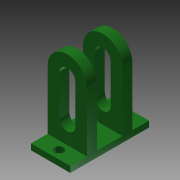
# Autodesk Inventor part: Tensioning Bracket
Saved by Autodesk Inventor 2015 SP1 (Build 190203100, 203)
## iProperties
Created: 2015-03-04
Part Number: Tensioning Bracket
Material: PC/ABS Plastic
Document SubType Name: Modeling
Designer: Andrew
Density: 0.357273 g/cm^3
Appearance: Smooth - Dark Forest Green
Author: Andrew
Autodesk Inventor part; units mm, degrees
ref_plane "YZ Plane" through (0, 0, 0) normal (1, 0, 0) x (0, 1, 0)
ref_plane "XZ Plane" through (0, 0, 0) normal (0, 1, 0) x (-1, 0, 0)
ref_plane "XY Plane" through (0, 0, 0) normal (0, 0, 1) x (1, 0, 0)
sketch "Sketch1" plane through (0, 0, 0) normal (0, 0, 1) x (1, 0, 0)
  line L0 (-10, -20) -> (10, -20)
  line L1 (10, -20) -> (10, 20)
  line L2 (10, 20) -> (-10, 20)
  line L3 (-10, 20) -> (-10, -20)
  line L4 (-10, -20) -> (10, 20) construction
  line L5 (10, -20) -> (-10, 20) construction
  line L6 (-10, 11.5) -> (10, 11.5)
  line L7 (10, 6.5) -> (-10, 6.5)
  line L8 (-10, -6.5) -> (10, -6.5)
  line L9 (10, -11.5) -> (-10, -11.5)
  line L10 (-4, 11.5) -> (-4, 6.5) construction
  line L11 (4, 6.5) -> (4, 11.5) construction
  line L12 (0, 28) -> (0, -28) construction
  line L13 (-14, 0) -> (14, 0) construction
  circle A0 centre (0, -15.75) radius 2.25
  circle A1 centre (0, 15.75) radius 2.25
  line L14 (-10, 15.75) -> (10, 15.75) construction
  point P0 (0, 0)
  dimension "d0" = 8
  dimension "d1" = 20
  dimension "d2" = 13
  dimension "d3" = 5
  dimension "d4" = 5
  dimension "d5" = 40
  dimension "d6" = 4.5
  constraints: 26 end point, 16 point on line, 7 perpendicular, 3 midpoint, 2 centre point, 2 horizontal, 2 parallel, 4 other
  measures "d0" distance between parallel lines of L11 L10
  measures "d1" distance between parallel lines of L3 L1
  measures "d2" distance between parallel lines of L8 L7
  measures "d3" distance between parallel lines of L7 L6
  measures "d4" distance between parallel lines of L9 L8
  measures "d5" distance between parallel lines of L0 L2
  measures "d6" diameter of A1
extrude "Extrusion1" add sketch "Sketch1" against normal blind 3
extrude "Extrusion2" add sketch "Sketch1" along normal blind 40 contours L3 L8 L1 L9 | L3 L6 L1 L7
sketch "Sketch2" plane through (-10, -11.5, 0) normal (0, -1, 0) x (1, 0, 0)
  line L0 (20, 0) -> (0, 0) projected
  line L1 (20, 0) -> (20, 40) projected
  line L2 (0, 40) -> (20, 40) projected
  line L3 (0, 0) -> (0, 40) projected
  line L4 (6, 34) -> (14, 34)
  line L5 (14, 34) -> (14, 6)
  line L6 (14, 6) -> (6, 6)
  line L7 (6, 6) -> (6, 34)
  line L8 (10, 48.6) -> (10, -11.6) projected
  point P0 (10, 0)
  dimension "d11" = 8
  dimension "d12" = 6
  dimension "d13" = 6
  constraints: 8 end point, 2 parallel, 1 horizontal, 1 perpendicular, 1 other
  measures "d11" distance between parallel lines of L5 L7
  measures "d12" distance between parallel lines of L2 L4
  measures "d13" distance between parallel lines of L0 L6
extrude "Extrusion3" cut sketch "Sketch2" against normal up to surface (23 mm away) contours L8 L4 L5 L6 | L6 L7 L4 L8
full round fillet "Fillet1" first side at (4, 8.1667, 24.6667) centre faces at (-1.3333, 8.1667, 34) second side at (-4, 8.1667, 15.3333)
full round fillet "Fillet2" first side at (4, 8.1667, 22.0001) centre faces at (1.3333, 8.1667, 6) second side at (-4, 8.1667, 14)
full round fillet "Fillet3" first side at (4, -9.8333, 24.6667) centre faces at (1.3333, -9.8333, 6) second side at (-4, -9.8333, 15.3333)
full round fillet "Fillet4" first side at (4, -8.1667, 26) centre faces at (1.3333, -8.1667, 34) second side at (-4, -9.8333, 17.9999)
full round fillet "Fillet5" first side at (10, -9.8333, 26.6667) centre faces at (3.3333, -9.8333, 40) second side at (-10, 9.8333, 26.6667)
full round fillet "Fillet6" first side at (10, 8.1667, 13.3333) centre faces at (-3.3333, 8.1667, 40) second side at (-10, 8.1667, 26.6667)
equation "\"d13\" = d12"
body "Solid1"
